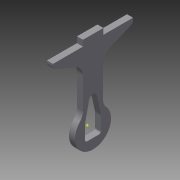
# Autodesk Inventor part: Camera Mount_B073113
Saved by Autodesk Inventor 2013 (Build 170138000, 138)
## iProperties
Created: 2013-05-28
Part Number: Camera Mount_B073113
Material: Generic
Document SubType Name: Modeling
Designer: Eric
Density: 1 g/cm^3
Author: Eric
Autodesk Inventor part; units mm, degrees
ref_plane "YZ Plane" through (0, 0, 0) normal (1, 0, 0) x (0, 1, 0)
ref_plane "XZ Plane" through (0, 0, 0) normal (0, 1, 0) x (-1, 0, 0)
ref_plane "XY Plane" through (0, 0, 0) normal (0, 0, 1) x (1, 0, 0)
sketch "Sketch1" plane through (0, 0, 0) normal (1, 0, 0) x (0, 1, 0)
  line L0 (-18.7654, 35.1522) -> (-8.7039, 30.9846)
  line L1 (8.7039, 30.9846) -> (18.7654, 35.1522)
  line L2 (-21, 41) -> (21, 41) construction
  line L3 (-5, 25.4414) -> (-5, 10.198)
  line L4 (5, 25.4414) -> (5, 10.198)
  arc A0 (-5, 25.4414) -> (-8.7039, 30.9846) centre (-11, 25.4414) ccw
  arc A1 (8.7039, 30.9846) -> (5, 25.4414) centre (11, 25.4414) ccw
  arc A2 (-6.6, 6.1188) -> (6.6, 6.1188) centre (0, 0) ccw
  arc A3 (-6.6, 6.1188) -> (-5, 10.198) centre (-11, 10.198) ccw
  arc A4 (5, 10.198) -> (6.6, 6.1188) centre (11, 10.198) ccw
  line L5 (4, 3.3563) -> (4, -3)
  line L6 (3, -4) -> (-3, -4)
  line L7 (-4, -3) -> (-4, 3.3563)
  line L8 (-4, 4) -> (4, -4) construction
  line L9 (4, 4) -> (-4, -4) construction
  arc A5 (1.9545, 13.4242) -> (-1.9545, 13.4242) centre (0, 13) ccw
  line L10 (0, 13) -> (0, 0) construction
  line L11 (-3.8635, 4.629) -> (-1.9545, 13.4242)
  line L12 (3.8635, 4.629) -> (1.9545, 13.4242)
  arc A6 (-3.8635, 4.629) -> (-4, 3.3563) centre (2, 3.3563) ccw
  arc A7 (4, 3.3563) -> (3.8635, 4.629) centre (-2, 3.3563) ccw
  arc A8 (-4, -3) -> (-3, -4) centre (-3, -3) ccw
  arc A9 (3, -4) -> (4, -3) centre (3, -3) ccw
  line L13 (-5, 38) -> (-5, 41)
  line L14 (5.2222, 41) -> (5.2222, 38)
  line L15 (-20, 38) -> (-5, 38)
  line L16 (5.2222, 38) -> (20, 38)
  line L17 (-20, 38) -> (-20, 37)
  line L18 (20, 38) -> (20, 37)
  circle A10 centre (0, 0) radius 46 construction
  arc A11 (-20, 37) -> (-18.7654, 35.1522) centre (-18, 37) ccw
  arc A12 (18.7654, 35.1522) -> (20, 37) centre (18, 37) ccw
  line L19 (-5, 40.9488) -> (5.2222, 40.9409)
  point P0 (-5, 29.4504)
  point P1 (5, 29.4504)
  point P2 (-5, 7.4833)
  point P3 (5, 7.4833)
  point P4 (0, 0)
  dimension "d25" = 10
  dimension "d32" = 6
  dimension "d33" = 6
  dimension "d68" = 18
  dimension "d69" = 6
  dimension "d75" = 8
  dimension "d76" = 8
  dimension "d77" = 4
  dimension "d78" = 13
  dimension "d79" = 6
  dimension "d80" = 1
  dimension "d82" = 46
  dimension "d84" = 38
  dimension "d85" = 3
  dimension "d86" = 5
  dimension "d87" = 20
  dimension "d88" = 40
  dimension "d90" = 2
  dimension "d93" = 1
  dimension "d94" = 1
  dimension "d95" = 22.5
  dimension "d96" = 22.5
  dimension "d97" = 4
  dimension "d98" = 4
  constraints: 40 end point, 26 point on circle, 22 tangent, 18 point on line, 13 centre point, 5 coincident, 4 equal radius, 4 parallel, 4 perpendicular, 3 horizontal, 3 midpoint, 2 vertical, 1 collinear
  measures "d25" distance between parallel lines of L3 L4
  measures "d32" radius of A0
  measures "d33" radius of A1
  measures "d68" diameter of A2
  measures "d69" radius of A3
  measures "d75" distance of L8.end L9.end
  measures "d76" distance of L9.end L8.start
  measures "d77" diameter of A5
  measures "d78" distance of L10.end L10.start
  measures "d79" radius of A6
  measures "d80" radius of A8
  measures "d82" radius of A10
  measures "d84" distance from line of A2.centre L15
  measures "d85" distance between parallel lines of L15 L2
  measures "d86" distance from line of L10.end L13
  measures "d87" distance from line of A2.centre L17
  measures "d88" distance between parallel lines of L17 L18
  measures "d90" radius of A11
  measures "d93" distance from line of L15 A11.centre
  measures "d94" distance from line of L16 A12.centre
  measures "d95" angle of L0 L15
  measures "d96" angle of L1 L16
  measures "d97" distance from line of A2.centre L6
  measures "d98" distance from line of L7 A2.centre
extrude "Extrusion6" add sketch "Sketch1" along normal blind 3
body "Solid6"
